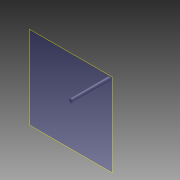
# Autodesk Inventor part: wheelAxel01
Saved by Autodesk Inventor 2013 (Build 170138000, 138)
## iProperties
Created: 2013-01-21
Part Number: wheelAxel01
Material: Stainless Steel
Document SubType Name: Modeling
Designer: Nano
Mass: 155.989 g
Surface Area: 63.3384 cm^2
Volume: 19.3056 cm^3
Density: 8.08 g/cm^3
Author: Nano
Autodesk Inventor part; units mm, degrees
note: some values were not read from the file. Chosen so that the rebuilt part matches the saved one: second side of "Extrusion1".
ref_plane "YZ Plane" through (0, 0, 0) normal (1, 0, 0) x (0, 1, 0)
ref_plane "XZ Plane" through (0, 0, 0) normal (0, 1, 0) x (-1, 0, 0)
ref_plane "XY Plane" through (0, 0, 0) normal (0, 0, 1) x (1, 0, 0)
ref_plane "Work Plane1" through (0, 0, -12.7) normal (0, 0, -1) x (-1, 0, 0)
sketch "Sketch1" plane through (0, 0, -12.7) normal (0, 0, -1) x (-1, 0, 0)
  circle A0 centre (0, 0) radius 5.9531
  point P0 (0, 0)
  dimension "d0" = 11.9062
  constraints: 1 centre point, 1 coincident
  measures "d0" diameter of A0
extrude "Extrusion1" add sketch "Sketch1" along normal blind 119.0625
body "Solid1"
